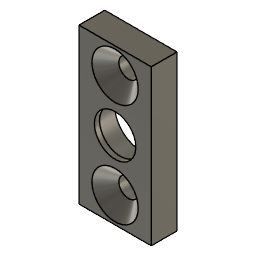
magnet body (Autodesk Fusion 360 design; units mm, degrees)
Autodesk Fusion 360 part; units mm, degrees
sketch "Sketch1" plane through (0, 0, 0) normal (0, 1, 0) x (1, 0, 0)
  circle A0 centre (0, 0) radius 5.075
  line L0 (-7, 15) -> (7, 15)
  line L1 (7, 15) -> (7, -15)
  line L2 (7, -15) -> (-7, -15)
  line L3 (-7, -15) -> (-7, 15)
  line L4 (-7, 15) -> (7, -15) construction
  line L5 (7, 15) -> (-7, -15) construction
  dimension "d1" = 10.15
  dimension "d2" = 7
  dimension "d3" = 30
  constraint coincident A0.centre origin
  constraint horizontal L0
  constraint perpendicular L0 L1
  constraint parallel L0 L2
  constraint parallel L1 L3
  constraint coincident L4 A0.centre
  constraint coincident L5 A0.centre
  measures "d1" diameter of A0
  measures "d2" distance of A0.centre L3
  measures "d3" distance of L0 L2
extrude "Extrude1" add sketch "Sketch1" along normal blind 5
sketch "Sketch2" plane through (0, 0, 0) normal (0, -1, 0) x (1, 0, 0)
  circle A0 centre (0, 0) radius 5.075
  line L0 (7, 15) -> (-7, 15)
  line L1 (-7, 15) -> (-7, -15)
  line L2 (-7, -15) -> (7, -15)
  line L3 (7, -15) -> (7, 15)
  line L4 (0, 15) -> (0, -15) construction
  line L5 (0, 0) -> (33.31, 0) construction
  circle A1 centre (0, 10) radius 1.875
  circle A2 centre (0, -10) radius 1.875
  dimension "d6" = 3.75
  constraint midpoint L0 L4.start
  constraint midpoint L2 L4.end
  constraint coincident A0.centre L5.start
  constraint perpendicular L4 L5
  constraint coincident L4 A1.centre
  constraint symmetric L5 A1 A2
  measures "d6" diameter of A1
extrude "Extrude2" cut sketch "Sketch2" against normal blind 31 contours A1 | A2
chamfer "Chamfer1" distance 2.6 angle 45 2 edges at (-1.7481, 0, 10.678) (-1.7481, 0, -9.322)
sketch "Sketch3" plane through (0, 0, 0) normal (0, -1, 0) x (1, 0, 0)
  line L0 (7, -15) -> (7, 15)
  line L1 (7, 15) -> (-7, 15)
  line L2 (-7, 15) -> (-7, -15)
  line L3 (-7, -15) -> (7, -15)
  circle A0 centre (0, 0) radius 5.075
  circle A1 centre (0, 0) radius 4
  circle A2 centre (0, 0) radius 5.075
  circle A3 centre (0, 10) radius 4.475
  circle A4 centre (0, -10) radius 4.475
  dimension "d10" = 8
  constraint concentric A0 A2
  constraint concentric A0 A1
  measures "d10" diameter of A1
extrude "Extrude3" add sketch "Sketch3" against normal blind 1 contours A0 A2
